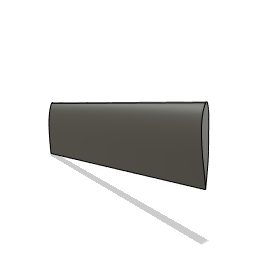
Zagi_Wing (Autodesk Fusion 360 design; units mm, degrees)
Autodesk Fusion 360 part; units mm, degrees
sketch "Skizze1" plane through (0, 0, 0) normal (1, 0, 0) x (0, 0, -1)
  line L0 (0, 0) -> (-45, 0) construction
  line L1 (-45, 0) -> (-45, -252.5) construction
  line L2 (-45, -252.5) -> (0, -252.5) construction
  line L3 (0, -252.5) -> (0, 0) construction
  line L4 (-14, -5) -> (-16.5, -247.5) construction
  line L5 (-16.1648, -214.9894) -> (-19.3648, -214.9564) construction
  line L6 (-16.0618, -204.9899) -> (-20.3618, -204.9456) construction
  line L7 (-15.9587, -194.9904) -> (-21.3087, -194.9353) construction
  line L8 (-15.8556, -184.991) -> (-22.1556, -184.926) construction
  line L9 (-15.7525, -174.9915) -> (-23.3525, -174.9131) construction
  line L10 (-15.6494, -164.992) -> (-24.8494, -164.8972) construction
  line L11 (-15.5463, -154.9926) -> (-25.7963, -154.8869) construction
  line L12 (-15.4432, -144.9931) -> (-26.9432, -144.8745) construction
  line L13 (-15.3401, -134.9936) -> (-27.6901, -134.8663) construction
  line L14 (-15.2371, -124.9942) -> (-28.4871, -124.8576) construction
  line L15 (-15.134, -114.9947) -> (-29.134, -114.8504) construction
  line L16 (-15.0309, -104.9952) -> (-29.5309, -104.8457) construction
  line L17 (-14.9278, -94.9957) -> (-29.7278, -94.8432) construction
  line L18 (-14.8247, -84.9963) -> (-29.8247, -84.8416) construction
  line L19 (-14.7216, -74.9968) -> (-30.2216, -74.837) construction
  line L20 (-14.6185, -64.9973) -> (-29.8685, -64.8401) construction
  line L21 (-14.5154, -54.9979) -> (-29.2154, -54.8463) construction
  line L22 (-14.4124, -44.9984) -> (-28.4124, -44.8541) construction
  line L23 (-14.3093, -34.9989) -> (-26.8093, -34.8701) construction
  line L24 (-14.2062, -24.9995) -> (-24.4562, -24.8938) construction
  line L25 (-14.1031, -15) -> (-22.1027, -14.9175) construction
  line L26 (-16.1648, -214.9894) -> (-12.8648, -215.0234) construction
  line L27 (-16.0618, -204.9899) -> (-12.1618, -205.0301) construction
  line L28 (-15.9587, -194.9904) -> (-16.0618, -194.9894) construction
  line L29 (-15.9587, -194.9904) -> (-10.2587, -195.0492) construction
  line L30 (-15.8556, -184.991) -> (-9.7556, -185.0539) construction
  line L31 (-15.7525, -174.9915) -> (-8.8525, -175.0626) construction
  line L32 (-15.6494, -164.992) -> (-8.1494, -165.0693) construction
  line L33 (-15.5463, -154.9926) -> (-7.5463, -155.075) construction
  line L34 (-15.4432, -144.9931) -> (-7.1932, -145.0781) construction
  line L35 (-14.5154, -54.9979) -> (-6.2654, -55.0829) construction
  line L36 (-14.4124, -44.9984) -> (-6.4124, -45.0809) construction
  line L37 (-14.3093, -34.9989) -> (-7.0593, -35.0737) construction
  line L38 (-14.2062, -24.9995) -> (-13.6374, -25.0053) construction
  line L39 (-13.6374, -25.0053) -> (-7.4374, -25.0692) construction
  line L40 (-14.1031, -15) -> (-9.1031, -15.0515) construction
  line L41 (-28.6876, -57.2976) -> (-28.6876, -53.2976) construction
  line L42 (-28.6876, -53.2976) -> (-31.6876, -53.2976) construction
  line L43 (-31.6876, -53.2976) -> (-31.6876, -57.2976) construction
  line L44 (-31.6876, -57.2976) -> (-28.6876, -57.2976) construction
  line L45 (-30, -107) -> (-30, -102) construction
  line L46 (-30, -102) -> (-35, -102) construction
  line L47 (-35, -102) -> (-35, -107) construction
  line L48 (-35, -107) -> (-30, -107) construction
  line L49 (-29, -158) -> (-29, -151) construction
  line L50 (-29, -151) -> (-35, -151) construction
  line L51 (-35, -151) -> (-35, -158) construction
  line L52 (-35, -158) -> (-29, -158) construction
  line L53 (-28, -208) -> (-28, -201) construction
  line L54 (-28, -201) -> (-33, -201) construction
  line L55 (-33, -201) -> (-33, -208) construction
  line L56 (-33, -208) -> (-28, -208) construction
  line L57 (-7.1932, -145.0781) -> (-6.2654, -55.0829)
  spline S0 degree 5 poles (-16.5443, -3.4105) (-16.8211, -3.8536) (-17.3625, -4.736) (-18.1376, -6.0481) (-19.0957, -7.7757) (-20.1593, -9.9029) (-21.0815, -12.0043) (-21.8605, -14.0867) (-22.504, -16.1568) (-23.0359, -18.2196) (-23.4929, -20.2782) (-23.9156, -22.3348) (-24.3408, -24.3908) (-24.7941, -26.4468) (-25.2807, -28.5038) (-25.7887, -30.5626) (-26.2966, -32.624) (-26.7804, -34.6888) (-27.2193, -36.7572) (-27.6034, -38.8295) (-27.9316, -40.9055) (-28.2087, -42.9849) (-28.4433, -45.0671) (-28.6445, -47.1516) (-28.8204, -49.2376) (-28.9776, -51.3247) (-29.1221, -53.4121) (-29.2588, -55.4996) (-29.3925, -57.587) (-29.5269, -59.6743) (-29.6644, -61.7617) (-29.8041, -63.8494) (-29.9416, -65.9377) (-30.0671, -68.0266) (-30.1669, -70.116) (-30.2275, -72.2058) (-30.2394, -74.2959) (-30.2002, -76.3859) (-30.1194, -78.476) (-30.0153, -80.566) (-29.9092, -82.6561) (-29.8206, -84.7462) (-29.762, -86.8365) (-29.7337, -88.9269) (-29.7276, -91.0175) (-29.7308, -93.1081) (-29.73, -95.1988) (-29.7152, -97.2894) (-29.6831, -99.38) (-29.6349, -101.4704) (-29.5741, -103.5608) (-29.5051, -105.651) (-29.431, -107.7412) (-29.3523, -109.8313) (-29.2681, -111.9213) (-29.1763, -114.0113) (-29.0744, -116.1012) (-28.9595, -118.1909) (-28.8296, -120.2801) (-28.6835, -122.3689) (-28.5222, -124.457) (-28.3491, -126.5447) (-28.1712, -128.6321) (-27.9968, -130.7198) (-27.8334, -132.808) (-27.6848, -134.897) (-27.5494, -136.9866) (-27.4168, -139.0763) (-27.2733, -141.1653) (-27.1052, -143.2529) (-26.9038, -145.3388) (-26.6696, -147.4231) (-26.4153, -149.5067) (-26.1586, -151.5908) (-25.9171, -153.6764) (-25.7028, -155.7641) (-25.5152, -157.8533) (-25.3402, -159.9425) (-25.1582, -162.03) (-24.9492, -164.1143) (-24.6988, -166.1949) (-24.4058, -168.2728) (-24.0811, -170.3505) (-23.742, -172.4306) (-23.408, -174.5149) (-23.0958, -176.6037) (-22.8144, -178.6943) (-22.5656, -180.7828) (-22.3465, -182.8652) (-22.1506, -184.9399) (-21.9702, -187.0089) (-21.7979, -189.0797) (-21.6273, -191.1616) (-21.453, -193.2617) (-21.2716, -195.3818) (-21.0819, -197.5137) (-20.885, -199.6378) (-20.6835, -201.732) (-20.4802, -203.7802) (-20.2776, -205.7795) (-20.0759, -207.7501) (-19.8737, -209.7369) (-19.6676, -211.7993) (-19.4535, -214.0033) (-19.2269, -216.4136) (-18.9833, -219.0843) (-18.7185, -222.0566) (-18.4289, -225.3612) (-18.111, -229.02) (-17.7622, -233.0473) (-17.3799, -237.4516) (-17.046, -241.2799) (-16.7794, -244.3231) (-16.5943, -246.4283) (-16.5, -247.5) knots 0 0 0 0 0 0 0.00909091 0.01818182 0.02727273 0.03636364 0.04545455 0.05454545 0.06363636 0.07272727 0.08181818 0.09090909 0.1 0.10909091 0.11818182 0.12727273 0.13636364 0.14545455 0.15454545 0.16363636 0.17272727 0.18181818 0.19090909 0.2 0.20909091 0.21818182 0.22727273 0.23636364 0.24545455 0.25454545 0.26363636 0.27272727 0.28181818 0.29090909 0.3 0.30909091 0.31818182 0.32727273 0.33636364 0.34545455 0.35454545 0.36363636 0.37272727 0.38181818 0.39090909 0.4 0.40909091 0.41818182 0.42727273 0.43636364 0.44545455 0.45454545 0.46363636 0.47272727 0.48181818 0.49090909 0.5 0.50909091 0.51818182 0.52727273 0.53636364 0.54545455 0.55454545 0.56363636 0.57272727 0.58181818 0.59090909 0.6 0.60909091 0.61818182 0.62727273 0.63636364 0.64545455 0.65454545 0.66363636 0.67272727 0.68181818 0.69090909 0.7 0.70909091 0.71818182 0.72727273 0.73636364 0.74545455 0.75454545 0.76363636 0.77272727 0.78181818 0.79090909 0.8 0.80909091 0.81818182 0.82727273 0.83636364 0.84545455 0.85454545 0.86363636 0.87272727 0.88181818 0.89090909 0.9 0.90909091 0.91818182 0.92727273 0.93636364 0.94545455 0.95454545 0.96363636 0.97272727 0.98181818 0.99090909 1 1 1 1 1 1 construction
  spline S1 degree 5 poles (-11.0768, -4.3255) (-10.9783, -4.7523) (-10.7883, -5.6039) (-10.5245, -6.8746) (-10.2108, -8.5556) (-9.8584, -10.6352) (-9.5182, -12.6938) (-9.1666, -14.7331) (-8.792, -16.756) (-8.4052, -18.7668) (-8.032, -20.7708) (-7.7032, -22.7731) (-7.4461, -24.7783) (-7.275, -26.7894) (-7.1808, -28.807) (-7.1379, -30.8297) (-7.1131, -32.8552) (-7.0742, -34.8809) (-6.998, -36.9048) (-6.8801, -38.926) (-6.7304, -40.9447) (-6.5672, -42.9618) (-6.4123, -44.9785) (-6.2859, -46.9958) (-6.2012, -49.0146) (-6.1655, -51.0351) (-6.1789, -52.6532) (-6.2129, -53.8677) (-6.2461, -54.6778) (-6.2654, -55.0829) knots 0 0 0 0 0 0 0.04 0.08 0.12 0.16 0.2 0.24 0.28 0.32 0.36 0.4 0.44 0.48 0.52 0.56 0.6 0.64 0.68 0.72 0.76 0.8 0.84 0.88 0.92 0.96 1 1 1 1 1 1 construction
  spline S2 degree 5 poles (-7.1932, -145.0781) (-7.1963, -145.5182) (-7.2054, -146.3982) (-7.2276, -147.7182) (-7.2744, -149.4781) (-7.3608, -151.6779) (-7.4725, -153.8775) (-7.6045, -156.0768) (-7.748, -158.2758) (-7.8912, -160.4742) (-8.024, -162.672) (-8.1418, -164.8692) (-8.2485, -167.066) (-8.3617, -169.2627) (-8.5041, -171.4599) (-8.6935, -173.6578) (-8.9345, -175.8564) (-9.2071, -178.055) (-9.4661, -180.2521) (-9.6638, -182.4467) (-9.7681, -184.6384) (-9.7802, -186.8281) (-9.7585, -189.0194) (-9.7928, -191.2162) (-9.9673, -193.4214) (-10.3297, -195.6342) (-10.851, -197.8484) (-11.4119, -200.0513) (-11.8781, -202.2292) (-12.1517, -204.3725) (-12.2472, -206.4778) (-12.3273, -208.5587) (-12.4479, -210.6717) (-12.6374, -212.8923) (-12.8897, -215.3048) (-13.1925, -217.9858) (-13.538, -220.9923) (-13.9229, -224.3658) (-14.3471, -228.1343) (-14.8123, -232.3149) (-15.3218, -236.9168) (-15.7677, -240.9379) (-16.1248, -244.1447) (-16.3732, -246.3674) (-16.5, -247.5) knots 0 0 0 0 0 0 0.025 0.05 0.075 0.1 0.125 0.15 0.175 0.2 0.225 0.25 0.275 0.3 0.325 0.35 0.375 0.4 0.425 0.45 0.475 0.5 0.525 0.55 0.575 0.6 0.625 0.65 0.675 0.7 0.725 0.75 0.775 0.8 0.825 0.85 0.875 0.9 0.925 0.95 0.975 1 1 1 1 1 1 construction
  line L58 (-14.8393, -232.6636) -> (-18.1607, -262.3364)
  line L59 (-19.6077, -212.1973) -> (-13.3923, -282.8027)
  line L60 (-11.4552, -194.987) -> (-12.8683, -215.0732)
  line L61 (-1.9731, 19.9133) -> (-31.1155, -26.7343)
  spline S3 degree 5 poles (-16.5443, -3.4105) (-17.3295, -4.6563) (-18.8399, -7.2958) (-20.9256, -11.6992) (-23.3461, -18.3995) (-25.772, -27.8197) (-27.6107, -37.862) (-28.8921, -48.1139) (-29.6745, -58.2875) (-30.0457, -68.2775) (-30.1052, -78.0926) (-29.9503, -87.8132) (-29.6617, -97.5423) (-29.2865, -107.3532) (-28.831, -117.258) (-28.278, -127.2333) (-27.6002, -137.235) (-26.7741, -147.2177) (-25.7961, -157.1525) (-24.6916, -167.0404) (-23.5035, -176.901) (-22.2843, -186.7656) (-21.0868, -196.6688) (-19.9545, -206.6405) (-18.9151, -216.6992) (-17.9841, -226.8553) (-17.3318, -235.0617) (-16.8954, -241.2629) (-16.6279, -245.4175) (-16.5, -247.5) knots 0 0 0 0 0 0 0.04 0.08 0.12 0.16 0.2 0.24 0.28 0.32 0.36 0.4 0.44 0.48 0.52 0.56 0.6 0.64 0.68 0.72 0.76 0.8 0.84 0.88 0.92 0.96 1 1 1 1 1 1
  spline S4 degree 5 poles (-6.2654, -55.0829) (-6.2551, -53.8837) (-6.2433, -51.5008) (-6.2525, -47.9728) (-6.3194, -43.363) (-6.5005, -37.7692) (-6.7888, -32.3606) (-7.1952, -27.1557) (-7.7282, -22.1696) (-8.3881, -17.4024) (-9.1672, -12.8412) (-9.8792, -9.3454) (-10.4601, -6.8044) (-10.8678, -5.1459) (-11.0768, -4.3255) knots 0 0 0 0 0 0 0.1 0.2 0.3 0.4 0.5 0.6 0.7 0.8 0.9 1 1 1 1 1 1
  spline S5 degree 5 poles (-7.1932, -145.0781) (-7.2173, -146.2089) (-7.2752, -148.5017) (-7.3916, -152.0346) (-7.6063, -156.9336) (-7.9754, -163.3751) (-8.4453, -170.1297) (-9.0128, -177.1772) (-9.6682, -184.4695) (-10.3943, -191.927) (-11.1701, -199.4539) (-11.9731, -206.9493) (-12.7822, -214.3188) (-13.5799, -221.4864) (-14.3555, -228.408) (-15.1031, -235.0639) (-15.6771, -240.1721) (-16.0938, -243.8827) (-16.3656, -246.3031) (-16.5, -247.5) knots 0 0 0 0 0 0 0.066667 0.133333 0.2 0.266667 0.333333 0.4 0.466667 0.533333 0.6 0.666667 0.733333 0.8 0.866667 0.933333 1 1 1 1 1 1
  arc A0 (-11.0768, -4.3255) -> (-16.5443, -3.4105) centre (-14, -5) ccw
  line L62 (-6.0886, 13.179) -> (-27, -20)
  point P0 (-14.1031, -15)
  point P1 (-14.2062, -24.9995)
  point P2 (-14.3093, -34.9989)
  point P3 (-14.4124, -44.9984)
  point P4 (-14.5154, -54.9979)
  point P5 (-14.6185, -64.9973)
  point P6 (-14.7216, -74.9968)
  point P7 (-14.8247, -84.9963)
  point P8 (-14.9278, -94.9957)
  point P9 (-15.0309, -104.9952)
  point P10 (-15.134, -114.9947)
  point P11 (-15.2371, -124.9942)
  point P12 (-15.3401, -134.9936)
  point P13 (-15.4432, -144.9931)
  point P14 (-15.5463, -154.9926)
  point P15 (-15.6494, -164.992)
  point P16 (-15.7525, -174.9915)
  point P17 (-15.8556, -184.991)
  point P18 (-15.9587, -194.9904)
  point P19 (-16.0618, -204.9899)
  point P20 (-16.1648, -214.9894)
  point P21 (-28.4124, -44.8541)
  point P22 (-29.7278, -94.8432)
  point P23 (-26.9432, -144.8745)
  point P24 (-21.3087, -194.9353)
  point P25 (-7.4374, -25.0692)
  point P26 (-8.8525, -175.0626)
  point P27 (-12.8683, -215.0732)
  dimension "d1" = 45
  dimension "d2" = 252.5
  dimension "d3" = 14
  dimension "d4" = 5
  dimension "d5" = 16.5
  dimension "d6" = 5
  dimension "d7" = 10
  dimension "d10" = 10
  dimension "d11" = 0
  dimension "d12" = 8
  dimension "d13" = 10.25
  dimension "d14" = 12.5
  dimension "d15" = 14
  dimension "d16" = 14.7
  dimension "d17" = 15.25
  dimension "d18" = 15.5
  dimension "d19" = 10
  dimension "d20" = 10
  dimension "d21" = 10
  dimension "d22" = 10
  dimension "d23" = 15
  dimension "d24" = 14.8
  dimension "d25" = 14.5
  dimension "d26" = 14
  dimension "d27" = 13.25
  dimension "d28" = 12.35
  dimension "d29" = 11.5
  dimension "d30" = 10.25
  dimension "d31" = 9.2
  dimension "d32" = 7.6
  dimension "d33" = 6.3
  dimension "d34" = 5.35
  dimension "d35" = 4.3
  dimension "d36" = 3.2
  dimension "d37" = 32.5124
  dimension "d38" = 5
  dimension "d39" = 6.2
  dimension "d40" = 7.25
  dimension "d41" = 8
  dimension "d42" = 8.25
  dimension "d44" = 8
  dimension "d45" = 7.5
  dimension "d46" = 6.9
  dimension "d47" = 6.1
  dimension "d48" = 5.7
  dimension "d49" = 3.9
  dimension "d50" = 3.3
  dimension "d51" = 6
  constraint horizontal L0
  constraint vertical L1
  constraint horizontal L2
  constraint vertical L3
  constraint coincident L0.start L3.end
  constraint coincident L4 P0
  constraint coincident P20 L5.start
  constraint perpendicular L4 L5
  constraint coincident P19 L6.start
  constraint perpendicular L4 L6
  constraint coincident P18 L7.start
  constraint perpendicular L4 L7
  constraint coincident P17 L8.start
  constraint perpendicular L4 L8
  constraint coincident P16 L9.start
  constraint perpendicular L4 L9
  constraint coincident P15 L10.start
  constraint perpendicular L4 L10
  constraint coincident P14 L11.start
  constraint perpendicular L4 L11
  constraint coincident P13 L12.start
  constraint perpendicular L4 L12
  constraint coincident P12 L13.start
  constraint perpendicular L4 L13
  constraint coincident P11 L14.start
  constraint perpendicular L4 L14
  constraint coincident P10 L15.start
  constraint perpendicular L4 L15
  constraint coincident P9 L16.start
  constraint perpendicular L4 L16
  constraint coincident P8 L17.start
  constraint perpendicular L4 L17
  constraint coincident P7 L18.start
  constraint perpendicular L4 L18
  constraint coincident P6 L19.start
  constraint perpendicular L4 L19
  constraint coincident P5 L20.start
  constraint perpendicular L4 L20
  constraint coincident P4 L21.start
  constraint perpendicular L4 L21
  constraint coincident P3 L22.start
  constraint perpendicular L4 L22
  constraint coincident P2 L23.start
  constraint perpendicular L4 L23
  constraint coincident P1 L24.start
  constraint perpendicular L4 L24
  constraint coincident P0 L25.start
  constraint perpendicular L4 L25
  constraint perpendicular L4 L26
  constraint perpendicular L4 L27
  constraint perpendicular L4 L28
  constraint perpendicular L4 L29
  constraint perpendicular L4 L30
  constraint perpendicular L4 L31
  constraint perpendicular L4 L32
  constraint perpendicular L4 L33
  constraint perpendicular L4 L34
  constraint perpendicular L4 L35
  constraint perpendicular L4 L36
  constraint perpendicular L4 L37
  constraint perpendicular L4 L38
  constraint perpendicular L4 L39
  constraint perpendicular L4 L40
  constraint parallel L4 L57
  constraint coincident L35.end L57
  constraint coincident L35.end L57.end
  constraint coincident L4.start A0.centre
  constraint coincident S0.start A0
  constraint midpoint L4.end L58
  constraint coincident L26.end L58
  constraint midpoint L4.end L59
  constraint coincident L5.end L59
  constraint midpoint L27.end L60
  constraint coincident L26.end L60
  constraint midpoint S0.start L61
  constraint tangent S0 A0
  constraint tangent S1 A0
  constraint coincident P21 L22.end
  constraint coincident P22 L17.end
  constraint coincident P23 L12.end
  constraint coincident P24 L7.end
  constraint coincident P25 L39.end
  constraint coincident P26 L31.end
  constraint coincident P27 L60.end
  constraint coincident S3 S0.start
  constraint midpoint S0.start L62
  measures "d1" distance of L0.start L0.end
  measures "d2" distance of L0.start L2.end
  measures "d3" horizontal distance of L0.start L4.start
  measures "d4" vertical distance of L0.start L4.start
  measures "d5" distance of L3 L4.end
  measures "d6" distance of L2 L4.end
  measures "d7" vertical distance of L4.start P0
  measures "d12" distance of L4 L25.end
  measures "d13" horizontal distance of P1 L24.end
  measures "d14" horizontal distance of P2 L23.end
  measures "d15" horizontal distance of P3 P21
  measures "d16" horizontal distance of P4 L21.end
  measures "d17" horizontal distance of P5 L20.end
  measures "d18" horizontal distance of P6 L19.end
  measures "d23" horizontal distance of P7 L18.end
  measures "d24" horizontal distance of P8 P22
  measures "d25" horizontal distance of P9 L16.end
  measures "d26" horizontal distance of P10 L15.end
  measures "d27" horizontal distance of P11 L14.end
  measures "d28" horizontal distance of P12 L13.end
  measures "d29" horizontal distance of P13 P23
  measures "d30" horizontal distance of P14 L11.end
  measures "d31" horizontal distance of P15 L10.end
  measures "d32" horizontal distance of P16 L9.end
  measures "d33" horizontal distance of P17 L8.end
  measures "d34" horizontal distance of P18 P24
  measures "d35" horizontal distance of P19 L6.end
  measures "d36" horizontal distance of P20 L5.end
  measures "d37" distance of L4.end L5
  measures "d38" horizontal distance of P0 L40.end
  measures "d39" horizontal distance of L38.end P25
  measures "d40" horizontal distance of P2 L37.end
  measures "d41" horizontal distance of P3 L36.end
  measures "d42" horizontal distance of P4 L35.end
  measures "d44" horizontal distance of P14 L33.end
  measures "d45" horizontal distance of P15 L32.end
  measures "d46" horizontal distance of P16 P26
  measures "d47" horizontal distance of P17 L30.end
  measures "d48" horizontal distance of P18 L29.end
  measures "d49" horizontal distance of P19 L27.end
  measures "d50" horizontal distance of P20 L26.end
  measures "d51" diameter of A0
ref_plane "Arbeitsebene1" through (-500, 0, 0) normal (1, 0, 0) x (0, 1, 0)
sketch "Skizze2" plane through (-500, 0, 0) normal (1, 0, 0) x (0, 0, -1)
  line L0 (0, -250) -> (-45, -250) construction
  line L1 (-45, -250) -> (-45, -400) construction
  line L2 (-45, -400) -> (0, -400) construction
  line L3 (0, -400) -> (0, -250) construction
  line L4 (-45, -252.5) -> (0, -252.5) construction
  line L5 (-45, 0) -> (-45, -252.5) construction
  line L6 (-14, -256.5) -> (-18, -395) construction
  line L7 (-14.2887, -266.4958) -> (-20.3861, -266.3197) construction
  line L8 (-14.5774, -276.4917) -> (-22.3741, -276.2665) construction
  line L9 (-14.8661, -286.4875) -> (-23.3625, -286.2421) construction
  line L10 (-15.1548, -296.4833) -> (-23.8511, -296.2322) construction
  line L11 (-15.4434, -306.4792) -> (-24.3397, -306.2222) construction
  line L12 (-15.7321, -316.475) -> (-24.2286, -316.2296) construction
  line L13 (-16.0208, -326.4708) -> (-24.2174, -326.2341) construction
  line L14 (-16.3095, -336.4667) -> (-23.2066, -336.2675) construction
  line L15 (-16.5982, -346.4625) -> (-21.9959, -346.3066) construction
  line L16 (-16.8869, -356.4583) -> (-21.485, -356.3255) construction
  line L17 (-17.1756, -366.4542) -> (-20.5742, -366.356) construction
  line L18 (-14.2887, -266.4958) -> (-10.2904, -266.6113) construction
  line L19 (-14.5774, -276.4917) -> (-10.2792, -276.6158) construction
  line L20 (-14.8661, -286.4875) -> (-10.168, -286.6232) construction
  line L21 (-15.1548, -296.4833) -> (-10.2568, -296.6248) construction
  line L22 (-15.4434, -306.4792) -> (-10.4455, -306.6235) construction
  line L23 (-16.0208, -326.4708) -> (-11.0229, -326.6152) construction
  line L24 (-16.3095, -336.4667) -> (-11.4115, -336.6081) construction
  line L25 (-16.5982, -346.4625) -> (-12.2, -346.5895) construction
  line L26 (-16.8869, -356.4583) -> (-12.6886, -356.5796) construction
  line L27 (-17.1756, -366.4542) -> (-13.5771, -366.5581) construction
  line L28 (-10.4455, -306.6235) -> (-11.0229, -326.6152)
  spline S0 degree 5 poles (-10.4455, -306.6235) (-10.4397, -306.2212) (-10.4275, -305.4166) (-10.4081, -304.2099) (-10.3797, -302.6013) (-10.3405, -300.5911) (-10.2983, -298.5814) (-10.2551, -296.572) (-10.2142, -294.5626) (-10.1803, -292.5529) (-10.1586, -290.5424) (-10.1531, -288.5309) (-10.1653, -286.5183) (-10.1926, -284.5049) (-10.2276, -282.4917) (-10.26, -280.4796) (-10.2805, -278.4694) (-10.2831, -276.4614) (-10.268, -274.4553) (-10.2445, -272.4492) (-10.2275, -270.441) (-10.2347, -268.4278) (-10.2839, -266.4071) (-10.39, -264.3768) (-10.5618, -262.3355) (-10.8044, -260.2826) (-11.0567, -258.6307) (-11.2788, -257.3864) (-11.4414, -256.5545) (-11.5264, -256.1379) knots 0 0 0 0 0 0 0.04 0.08 0.12 0.16 0.2 0.24 0.28 0.32 0.36 0.4 0.44 0.48 0.52 0.56 0.6 0.64 0.68 0.72 0.76 0.8 0.84 0.88 0.92 0.96 1 1 1 1 1 1 construction
  spline S1 degree 5 poles (-18, -395) (-17.824, -393.9501) (-17.4795, -391.8887) (-16.9855, -388.9118) (-16.3722, -385.1733) (-15.6819, -380.8864) (-15.0683, -376.9846) (-14.5317, -373.4605) (-14.0713, -370.2977) (-13.685, -367.4665) (-13.3693, -364.9213) (-13.1182, -362.5945) (-12.9236, -360.4035) (-12.775, -358.2666) (-12.66, -356.1148) (-12.5638, -353.9076) (-12.4703, -351.6415) (-12.3642, -349.3347) (-12.2344, -347.0158) (-12.076, -344.7115) (-11.8938, -342.4332) (-11.7, -340.1788) (-11.5097, -337.9389) (-11.3387, -335.7009) (-11.1986, -333.4543) (-11.0959, -331.1935) (-11.0461, -329.3711) (-11.0273, -327.9963) (-11.023, -327.0761) (-11.0229, -326.6152) knots 0 0 0 0 0 0 0.04 0.08 0.12 0.16 0.2 0.24 0.28 0.32 0.36 0.4 0.44 0.48 0.52 0.56 0.6 0.64 0.68 0.72 0.76 0.8 0.84 0.88 0.92 0.96 1 1 1 1 1 1 construction
  spline S2 degree 5 poles (-18, -395) (-18.0737, -394.0045) (-18.2203, -392.0491) (-18.4372, -389.2226) (-18.7207, -385.6673) (-19.0654, -381.5776) (-19.3999, -377.8383) (-19.7231, -374.4399) (-20.0334, -371.3665) (-20.3281, -368.5933) (-20.6039, -366.085) (-20.8559, -363.7938) (-21.0782, -361.658) (-21.2658, -359.6116) (-21.4166, -357.5928) (-21.533, -355.5528) (-21.625, -353.466) (-21.7097, -351.3324) (-21.8068, -349.1673) (-21.9347, -346.9928) (-22.1071, -344.8298) (-22.3281, -342.6877) (-22.5924, -340.565) (-22.888, -338.4541) (-23.1974, -336.3449) (-23.5001, -334.2288) (-23.7739, -332.1033) (-23.9985, -329.9697) (-24.1593, -327.8315) (-24.2503, -325.6932) (-24.2787, -323.5578) (-24.2655, -321.4257) (-24.2377, -319.2961) (-24.2205, -317.1674) (-24.231, -315.0379) (-24.2688, -312.9067) (-24.3175, -310.7741) (-24.3539, -308.6409) (-24.3554, -306.508) (-24.3079, -304.3764) (-24.2144, -302.2463) (-24.0897, -300.1178) (-23.954, -297.9904) (-23.8259, -295.8636) (-23.716, -293.7366) (-23.6215, -291.6088) (-23.5315, -289.4795) (-23.4312, -287.3488) (-23.3061, -285.2172) (-23.1468, -283.0865) (-22.9505, -280.9589) (-22.717, -278.837) (-22.4471, -276.7223) (-22.1397, -274.615) (-21.789, -272.5133) (-21.3853, -270.4133) (-20.9173, -268.3103) (-20.3735, -266.1996) (-19.7442, -264.077) (-19.0231, -261.9399) (-18.2066, -259.7866) (-17.4756, -258.0504) (-16.8833, -256.7406) (-16.469, -255.8639) (-16.2569, -255.4247) knots 0 0 0 0 0 0 0.01666667 0.03333333 0.05 0.06666667 0.08333333 0.1 0.11666667 0.13333333 0.15 0.16666667 0.18333333 0.2 0.21666667 0.23333333 0.25 0.26666667 0.28333333 0.3 0.31666667 0.33333333 0.35 0.36666667 0.38333333 0.4 0.41666667 0.43333333 0.45 0.46666667 0.48333333 0.5 0.51666667 0.53333333 0.55 0.56666667 0.58333333 0.6 0.61666667 0.63333333 0.65 0.66666667 0.68333333 0.7 0.71666667 0.73333333 0.75 0.76666667 0.78333333 0.8 0.81666667 0.83333333 0.85 0.86666667 0.88333333 0.9 0.91666667 0.93333333 0.95 0.96666667 0.98333333 1 1 1 1 1 1 construction
  spline S3 degree 5 poles (-18, -395) (-18.2218, -392.7777) (-18.656, -388.3998) (-19.2791, -382.0328) (-20.0534, -373.9448) (-20.9254, -364.5089) (-21.7, -355.7454) (-22.3752, -347.638) (-22.9502, -340.146) (-23.4249, -333.1961) (-23.8017, -326.6673) (-24.0843, -320.3979) (-24.2736, -314.2218) (-24.364, -307.9989) (-24.3407, -301.6448) (-24.1746, -295.1699) (-23.8267, -288.6629) (-23.2564, -282.2524) (-22.4278, -276.0771) (-21.3179, -270.2524) (-19.924, -264.8391) (-18.5885, -260.8559) (-17.4681, -258.0646) (-16.6693, -256.2902) (-16.2569, -255.4247) knots 0 0 0 0 0 0 0.05 0.1 0.15 0.2 0.25 0.3 0.35 0.4 0.45 0.5 0.55 0.6 0.65 0.7 0.75 0.8 0.85 0.9 0.95 1 1 1 1 1 1
  spline S4 degree 5 poles (-18, -395) (-17.7408, -393.4753) (-17.2324, -390.4393) (-16.5004, -385.9252) (-15.5864, -379.9877) (-14.5544, -372.7107) (-13.6437, -365.5929) (-12.8658, -358.6493) (-12.2295, -351.8914) (-11.7334, -345.3172) (-11.3683, -338.915) (-11.1734, -333.9207) (-11.0785, -330.2422) (-11.0377, -327.8193) (-11.0229, -326.6152) knots 0 0 0 0 0 0 0.1 0.2 0.3 0.4 0.5 0.6 0.7 0.8 0.9 1 1 1 1 1 1
  spline S5 degree 5 poles (-10.4455, -306.6235) (-10.4316, -305.4322) (-10.4048, -303.0646) (-10.3672, -299.5583) (-10.3227, -294.9752) (-10.2785, -289.4103) (-10.2514, -284.0265) (-10.2519, -278.8427) (-10.2967, -273.8752) (-10.4111, -269.1266) (-10.6265, -264.5872) (-10.9054, -261.1137) (-11.1865, -258.5933) (-11.4075, -256.9502) (-11.5264, -256.1379) knots 0 0 0 0 0 0 0.1 0.2 0.3 0.4 0.5 0.6 0.7 0.8 0.9 1 1 1 1 1 1
  arc A0 (-11.5264, -256.1379) -> (-16.2569, -255.4247) centre (-14, -256.5) ccw
  point P0 (-14, -256.5)
  point P1 (-14.2887, -266.4958)
  point P2 (-14.2887, -266.4958)
  point P3 (-14.2887, -266.4958)
  point P4 (-14.5774, -276.4917)
  point P5 (-14.5774, -276.4917)
  point P6 (-14.5774, -276.4917)
  point P7 (-14.8661, -286.4875)
  point P8 (-14.8661, -286.4875)
  point P9 (-14.8661, -286.4875)
  point P10 (-15.1548, -296.4833)
  point P11 (-15.1548, -296.4833)
  point P12 (-15.1548, -296.4833)
  point P13 (-15.4434, -306.4792)
  point P14 (-15.4434, -306.4792)
  point P15 (-15.4434, -306.4792)
  point P16 (-15.7321, -316.475)
  point P17 (-15.7321, -316.475)
  point P18 (-15.7321, -316.475)
  point P19 (-16.0208, -326.4708)
  point P20 (-16.0208, -326.4708)
  point P21 (-16.0208, -326.4708)
  point P22 (-16.3095, -336.4667)
  point P23 (-16.3095, -336.4667)
  point P24 (-16.3095, -336.4667)
  point P25 (-16.5982, -346.4625)
  point P26 (-16.5982, -346.4625)
  point P27 (-16.5982, -346.4625)
  point P28 (-16.8869, -356.4583)
  point P29 (-16.8869, -356.4583)
  point P30 (-16.8869, -356.4583)
  point P31 (-17.1756, -366.4542)
  point P32 (-17.1756, -366.4542)
  point P33 (-17.1756, -366.4542)
  point P34 (-23.2066, -336.2675)
  point P35 (-24.3397, -306.2222)
  point P36 (-22.3741, -276.2665)
  point P37 (-12.6886, -356.5796)
  point P38 (-10.2792, -276.6158)
  dimension "d53" = 150
  dimension "d54" = 250
  dimension "d55" = 14
  dimension "d56" = 4
  dimension "d57" = 18
  dimension "d58" = 5
  dimension "d59" = 5
  dimension "d62" = 10
  dimension "d63" = 0
  dimension "d65" = 6.1
  dimension "d66" = 7.8
  dimension "d67" = 8.5
  dimension "d68" = 8.7
  dimension "d69" = 8.9
  dimension "d70" = 8.5
  dimension "d71" = 8.2
  dimension "d72" = 6.9
  dimension "d73" = 5.4
  dimension "d74" = 4.6
  dimension "d75" = 3.4
  dimension "d76" = 4
  dimension "d77" = 4.3
  dimension "d78" = 4.7
  dimension "d79" = 4.9
  dimension "d80" = 5
  dimension "d82" = 4.9
  dimension "d83" = 4.4
  dimension "d84" = 4.2
  dimension "d85" = 3.6
  constraint horizontal L0
  constraint vertical L1
  constraint horizontal L2
  constraint vertical L3
  constraint equal L0 L4
  constraint collinear L1 L5
  constraint coincident P0 L6.start
  constraint coincident P3 P2
  constraint perpendicular L6 L7
  constraint coincident P6 P5
  constraint perpendicular L6 L8
  constraint coincident P9 P8
  constraint perpendicular L6 L9
  constraint coincident P12 P11
  constraint perpendicular L6 L10
  constraint coincident P15 P14
  constraint perpendicular L6 L11
  constraint coincident P18 P17
  constraint perpendicular L6 L12
  constraint coincident P21 P20
  constraint perpendicular L6 L13
  constraint coincident P24 P23
  constraint perpendicular L6 L14
  constraint coincident P27 P26
  constraint perpendicular L6 L15
  constraint coincident P30 P29
  constraint perpendicular L6 L16
  constraint coincident P33 P32
  constraint perpendicular L6 L17
  constraint perpendicular L6 L18
  constraint perpendicular L6 L19
  constraint perpendicular L6 L20
  constraint perpendicular L6 L21
  constraint perpendicular L6 L22
  constraint perpendicular L6 L23
  constraint perpendicular L6 L24
  constraint perpendicular L6 L25
  constraint perpendicular L6 L26
  constraint perpendicular L6 L27
  constraint equal L22 L23
  constraint coincident P34 L14.end
  constraint coincident P35 L11.end
  constraint coincident P36 L8.end
  constraint coincident P37 L26.end
  constraint coincident P38 L19.end
  constraint tangent S3 A0
  constraint tangent S5 A0
  measures "d53" distance of L0.start L2.end
  measures "d54" distance of L0 L5.start
  measures "d55" distance of L3 P0
  measures "d56" distance of L4 P0
  measures "d57" distance of L3 L6.end
  measures "d58" distance of L2 L6.end
  measures "d59" diameter of A0
  measures "d65" distance of P3 L7.end
  measures "d66" distance of P6 P36
  measures "d67" distance of P9 L9.end
  measures "d68" distance of P12 L10.end
  measures "d69" distance of P15 P35
  measures "d70" distance of P18 L12.end
  measures "d71" distance of P21 L13.end
  measures "d72" distance of P24 P34
  measures "d73" distance of P27 L15.end
  measures "d74" distance of P30 L16.end
  measures "d75" distance of P33 L17.end
  measures "d76" distance of P3 L18.end
  measures "d77" distance of P6 P38
  measures "d78" distance of P9 L20.end
  measures "d79" distance of P12 L21.end
  measures "d80" distance of P15 L22.end
  measures "d82" distance of P24 L24.end
  measures "d83" distance of P27 L25.end
  measures "d84" distance of P30 P37
  measures "d85" distance of P33 L27.end
loft "Erhebung1" add profiles "Skizze1", "Skizze2" section 1 section 2
